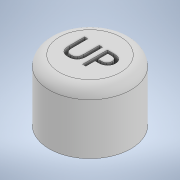
# Autodesk Inventor part: UP Button
Saved by Autodesk Inventor 2021 (Build 250183000, 183)
## iProperties
Created: 2021-03-30
Part Number: UP Button
Material: Generic
Document SubType Name: Modeling
Designer: eng1-177
Density: 1 g/cm^3
Appearance: Default
Author: eng1-177
Autodesk Inventor part; units mm, degrees
ref_plane "YZ Plane" through (0, 0, 0) normal (1, 0, 0) x (0, 1, 0)
ref_plane "XZ Plane" through (0, 0, 0) normal (0, 1, 0) x (-1, 0, 0)
ref_plane "XY Plane" through (0, 0, 0) normal (0, 0, 1) x (1, 0, 0)
sketch "Sketch1" plane through (0, 0, 0) normal (0, 1, 0) x (-1, 0, 0)
  circle A0 centre (0, 0) radius 10
  dimension "d0" = 20
  constraints: 1 centre point, 1 coincident
  measures "d0" diameter of A0
extrude "Extrusion1" add sketch "Sketch1" along normal blind 15
fillet "Fillet1" radius 2.5 1 edges at (10, 15, 0)
sketch "Sketch2" plane through (0, 15, 0) normal (0, 1, 0) x (1, 0, 0)
  line L0 (-4.9845, 3.1153) -> (3.7384, 3.1153) construction
  line L1 (3.7384, 3.1153) -> (3.7384, -3.4029) construction
  line L2 (3.7384, -3.4029) -> (-4.9845, -3.4029) construction
  line L3 (-4.9845, -3.4029) -> (-4.9845, 3.1153) construction
  spline S0 degree 2 poles (-2.236, -3.1132) (-2.7748, -3.1132) (-3.5756, -2.8315) (-3.8574, -2.5497) knots 0 0 0 1 2 2 2
  spline S1 degree 2 poles (-3.8574, -2.5497) (-4.1787, -2.2333) (-4.4407, -1.3435) (-4.4407, -0.691) knots 0 0 0 1 2 2 2
  line L4 (-4.4407, -0.691) -> (-4.4407, 3.1153)
  line L5 (-4.4407, 3.1153) -> (-3.63, 3.1153)
  line L6 (-3.63, 3.1153) -> (-3.63, -0.691)
  spline S2 degree 2 poles (-3.63, -0.691) (-3.63, -1.1162) (-3.5213, -1.6896) (-3.368, -1.9219) knots 0 0 0 1 2 2 2
  spline S3 degree 2 poles (-3.368, -1.9219) (-3.2049, -2.1691) (-2.6414, -2.4212) (-2.236, -2.4212) knots 0 0 0 1 2 2 2
  spline S4 degree 2 poles (-2.236, -2.4212) (-1.8554, -2.4212) (-1.2622, -2.1691) (-1.0991, -1.9219) knots 0 0 0 1 2 2 2
  spline S5 degree 2 poles (-1.0991, -1.9219) (-0.9458, -1.6896) (-0.8371, -1.1211) (-0.8371, -0.7108) knots 0 0 0 1 2 2 2
  line L7 (-0.8371, -0.7108) -> (-0.8371, 3.1153)
  line L8 (-0.8371, 3.1153) -> (-0.0264, 3.1153)
  line L9 (-0.0264, 3.1153) -> (-0.0264, -0.691)
  spline S6 degree 2 poles (-0.0264, -0.691) (-0.0264, -1.3287) (-0.2834, -2.2383) (-0.6097, -2.5497) knots 0 0 0 1 2 2 2
  spline S7 degree 2 poles (-0.6097, -2.5497) (-0.9013, -2.8364) (-1.6725, -3.1132) (-2.236, -3.1132) knots 0 0 0 1 2 2 2
  spline S8 degree 2 poles (4.9911, 1.2764) (4.9911, 0.8809) (4.7093, 0.1691) (4.4572, -0.0781) knots 0 0 0 1 2 2 2
  spline S9 degree 2 poles (4.4572, -0.0781) (4.1408, -0.3895) (3.2856, -0.7108) (2.6331, -0.7108) knots 0 0 0 1 2 2 2
  line L10 (2.6331, -0.7108) -> (1.946, -0.7108)
  line L11 (1.946, -0.7108) -> (1.946, -2.9847)
  line L12 (1.946, -2.9847) -> (1.1353, -2.9847)
  line L13 (1.1353, -2.9847) -> (1.1353, 3.1153)
  line L14 (1.1353, 3.1153) -> (2.6677, 3.1153)
  spline S10 degree 2 poles (2.6677, 3.1153) (3.2115, 3.1153) (3.9727, 2.9373) (4.2644, 2.7347) knots 0 0 0 1 2 2 2
  spline S11 degree 2 poles (4.2644, 2.7347) (4.6055, 2.5023) (4.9911, 1.7856) (4.9911, 1.2764) knots 0 0 0 1 2 2 2
  spline S12 degree 2 poles (4.1458, 1.2517) (4.1458, 1.568) (3.9283, 2.0327) (3.7058, 2.181) knots 0 0 0 1 2 2 2
  spline S13 degree 2 poles (3.7058, 2.181) (3.513, 2.3095) (2.9989, 2.4133) (2.6183, 2.4133) knots 0 0 0 1 2 2 2
  line L15 (2.6183, 2.4133) -> (1.946, 2.4133)
  line L16 (1.946, 2.4133) -> (1.946, -0.0187)
  line L17 (1.946, -0.0187) -> (2.4996, -0.0187)
  spline S14 degree 2 poles (2.4996, -0.0187) (2.994, -0.0187) (3.602, 0.1394) (3.7997, 0.3471) knots 0 0 0 1 2 2 2
  spline S15 degree 2 poles (3.7997, 0.3471) (3.9826, 0.53) (4.1458, 0.96) (4.1458, 1.2517) knots 0 0 0 1 2 2 2
  point P0 (0, 0)
  constraints: 2 other
extrude "Extrusion2" cut sketch "Sketch2" against normal blind 5
sketch "Sketch3" plane through (0, 0, 0) normal (0, -1, 0) x (1, 0, 0)
  circle A0 centre (0, 0) radius 7.5
  constraints: 1 centre point, 1 coincident
extrude "Extrusion3" cut sketch "Sketch3" against normal blind 2.5
body "Solid1"
